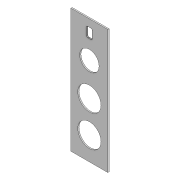
# Autodesk Inventor part: Front
Saved by Autodesk Inventor 2021.3 (Build 253353000, 353)
## iProperties
Created: 2021-11-26
Part Number: Front
Material: Generic
Document SubType Name: Modeling
Designer: wbrooks
Density: 1 g/cm^3
Appearance: Default
Author: wbrooks
Autodesk Inventor part; units mm, degrees
ref_plane "YZ Plane" through (0, 0, 0) normal (1, 0, 0) x (0, 1, 0)
ref_plane "XZ Plane" through (0, 0, 0) normal (0, 1, 0) x (-1, 0, 0)
ref_plane "XY Plane" through (0, 0, 0) normal (0, 0, 1) x (1, 0, 0)
sketch "Sketch1" plane through (0, 0, 0) normal (0, 0, 1) x (1, 0, 0)
  line L0 (180.975, 609.6) -> (-180.975, 609.6)
  line L1 (-180.975, 609.6) -> (-180.975, -609.6)
  line L2 (-180.975, -609.6) -> (180.975, -609.6)
  line L3 (180.975, -609.6) -> (180.975, 609.6)
  line L4 (180.975, 609.6) -> (-180.975, -609.6) construction
  line L5 (-180.975, 609.6) -> (180.975, -609.6) construction
  line L6 (0, 609.6) -> (0, -609.6)
  line L7 (-15.875, 537.21) -> (15.875, 537.21)
  line L8 (28.575, 524.51) -> (28.575, 453.39)
  line L9 (15.875, 440.69) -> (-15.875, 440.69)
  line L10 (-28.575, 453.39) -> (-28.575, 524.51)
  line L11 (-28.575, 537.21) -> (28.575, 440.69) construction
  line L12 (28.575, 537.21) -> (-28.575, 440.69) construction
  circle A0 centre (0, -381) radius 114.3
  circle A1 centre (0, -69.85) radius 114.3
  circle A2 centre (0, 254) radius 95.25
  arc A3 (-28.575, 453.39) -> (-15.875, 440.69) centre (-15.875, 453.39) ccw
  arc A4 (15.875, 440.69) -> (28.575, 453.39) centre (15.875, 453.39) ccw
  arc A5 (-15.875, 537.21) -> (-28.575, 524.51) centre (-15.875, 524.51) ccw
  arc A6 (28.575, 524.51) -> (15.875, 537.21) centre (15.875, 524.51) ccw
  point P0 (0, 0)
  point P1 (0, 488.95)
  dimension "d2" = 361.95
  dimension "d3" = 1219.2
  dimension "d4" = 120.65
  dimension "d6" = 990.6
  dimension "d7" = 679.45
  dimension "d8" = 228.6
  dimension "d9" = 228.6
  dimension "d11" = 190.5
  dimension "d12" = 355.6
  dimension "d13" = 96.52
  dimension "d14" = 57.15
  dimension "d16" = 12.7
  constraints: 26 end point, 11 point on line, 8 point on circle, 8 tangent, 7 centre point, 6 midpoint, 4 parallel, 3 equal radius, 2 horizontal, 2 perpendicular
  measures "d2" distance of L0.start L0.end
  measures "d3" distance of L2.end L0.start
  measures "d4" distance from line of L0 point (0, 488.95)
  measures "d6" distance from line of L0 A0.centre
  measures "d7" distance from line of L0 A1.centre
  measures "d8" diameter of A1
  measures "d9" diameter of A0
  measures "d11" diameter of A2
  measures "d12" distance from line of L0 A2.centre
  measures "d13" distance of L12.start L11.end
  measures "d14" distance of L11.start L12.start
  measures "d16" radius of A3
extrude "Extrusion1" add sketch "Sketch1" along normal mid plane 11.9062 contours L3 L2 L6 A0 A1 A2 L9 A4 L8 A6 L7 L0 | L6 L7 A5 L10 A3 L9 A2 A1 A0 L2 L1 L0
body "Solid1"
